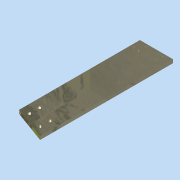
# Autodesk Inventor part: saule
Saved by Autodesk Inventor 2021 (Build 250183000, 183)
## iProperties
Created: 2024-03-13
Part Number: saule
Material: Generic
Document SubType Name: Modeling
Designer: Nokia
Density: 1 g/cm^3
Appearance: Plate - Blue
Mass: 377.9 g
Surface Area: 871.548 cm^2
Volume: 377.9 cm^3
Author: Nokia
Autodesk Inventor part; units mm, degrees
ref_plane "YZ Plane" through (0, 0, 0) normal (1, 0, 0) x (0, 1, 0)
ref_plane "XZ Plane" through (0, 0, 0) normal (0, 1, 0) x (-1, 0, 0)
ref_plane "XY Plane" through (0, 0, 0) normal (0, 0, 1) x (1, 0, 0)
sketch "Sketch1" plane through (0, 0, 0) normal (0, 0, 1) x (1, 0, 0)
  line L0 (-50, -30) -> (-50, -20)
  line L1 (-50, -20) -> (50, -20)
  line L2 (50, -20) -> (50, -30)
  line L3 (50, -30) -> (-50, -30)
  point P0 (0, 0)
  dimension "d0" = 100
  dimension "d3" = 10
  constraints: 8 end point, 2 perpendicular, 1 vertical
  measures "d0" distance of L0.end L1.end
  measures "d3" distance of L1.end L2.end
extrude "Extrusion1" add sketch "Sketch1" along normal blind 400
sketch "Sketch3" plane through (-50, -20, 0) normal (0, 1, 0) x (1, 0, 0)
  line L0 (100, -400) -> (0, -400) projected
  line L1 (100, 0) -> (100, -400) projected
  line L2 (100, -400) -> (0, -363.603)
  line L3 (0, -400) -> (100, -400)
  line L4 (0, -400) -> (0, -363.603)
  line L5 (0, 0) -> (0, -400) projected
  point P0 (50, 0)
  constraints: 6 end point, 1 collinear, 1 point on line
extrude "Extrusion2" cut sketch "Sketch3" against normal through all
sketch "Sketch4" plane through (-50, -20, 0) normal (0, 1, 0) x (1, 0, 0)
  line L0 (0, -363.603) -> (100, -400) projected
  line L1 (100, 0) -> (100, -400) projected
  line L2 (100, -400) -> (0, -363.603)
  line L3 (100, -340) -> (50, -321.8015)
  line L4 (0, 0) -> (0, -363.603) projected
  line L5 (0, -303.603) -> (0, -363.603)
  line L6 (75, -360.9007) -> (50, -351.8015)
  line L7 (100, -340) -> (100, -370)
  line L8 (50, -366.8015) -> (50, -336.8015)
  circle A0 centre (75, -345.9007) radius 5
  line L9 (100, -355) -> (75, -345.9007)
  line L10 (50, -336.8015) -> (25, -327.7022)
  line L11 (25, -327.7022) -> (25, -357.7022)
  circle A1 centre (25, -327.7022) radius 5
  line L12 (75, -390.9007) -> (75, -375.9007)
  line L13 (75, -350.9007) -> (75, -330.9007)
  circle A2 centre (75, -375.9007) radius 5
  circle A3 centre (25, -357.7022) radius 5
  line L14 (25, -357.7022) -> (50, -366.8015)
  line L15 (75, -375.9007) -> (100, -385)
  point P0 (50, 0)
  dimension "d26" = 10
  dimension "d27" = 10
  dimension "d28" = 10
  dimension "d36" = 25
  dimension "d37" = 26.6044
  dimension "d38" = 30
  dimension "d39" = 30
  dimension "d40" = 25
  dimension "d41" = 25
  dimension "d42" = 25
  dimension "d44" = 70
  dimension "d45" = 70
  dimension "d46" = 70
  dimension "d47" = 110
  dimension "d48" = 15
  constraints: 26 end point, 4 point on line, 3 centre point, 3 collinear, 3 midpoint, 2 parallel, 1 coincident, 1 vertical alignment, 2 other
  measures "d27" diameter of A1
  measures "d28" diameter of A2
  measures "d36" distance between parallel lines of L8 L12
  measures "d37" distance of L6.start L6.end
  measures "d38" distance of L8.start L8.end
  measures "d39" distance of L10.end L11.end
  measures "d40" horizontal distance of L12.end L15.end
  measures "d41" horizontal distance of L9.start L9.end
  measures "d42" horizontal distance of L11.end L8.start
  measures "d44" angle of L12 L15
  measures "d45" angle of L13 L9
  measures "d46" angle of L8 L6
  measures "d47" angle of L10 L8
  measures "d48" distance of L12.start L12.end
hole "Hole2" at (25, -20, 375.9007) at (25, -20, 345.9007) at (-25, -20, 357.7022) at (-25, -20, 327.7022) direction (0, -1, 0) diameter 10 end through all
sketch "Sketch5" plane through (-50, -30, 0) normal (0, -1, 0) x (1, 0, 0)
  line L0 (0, 0) -> (0, 363.603) projected
  line L1 (0, 0) -> (50, 0)
  line L2 (0, 0) -> (100, 0) projected
  line L3 (50, 0) -> (50, 10)
  circle A0 centre (25, 10) radius 5
  line L4 (50, 10) -> (50, 20)
  line L5 (50, 20) -> (67.2087, 20)
  circle A1 centre (75, 10) radius 5
  circle A2 centre (25, 30) radius 5
  circle A3 centre (75, 30) radius 5
  dimension "d49" = 10
  dimension "d50" = 10
  dimension "d51" = 10
  constraints: 8 end point, 4 centre point, 3 perpendicular, 3 symmetric about line, 1 collinear, 3 other
  measures "d49" distance of L1.end L3.end
  measures "d50" diameter of A0
  measures "d51" distance of L3.end L4.end
hole "Hole3" at (25, -30, 10) at (25, -30, 30) at (-25, -30, 10) at (-25, -30, 30) direction (0, 1, 0) diameter 6.647 end through all thread size "M8x1.25" class "6H" standard "ISO Metric profile"
body "Solid1"
